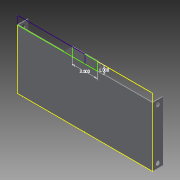
# Autodesk Inventor part: 4barFrontPlate
Saved by Autodesk Inventor 2015 SP1 (Build 190203100, 203)
## iProperties
Created: 2015-02-16
Part Number: 4barFrontPlate
Material: Generic
Document SubType Name: Modeling
Designer: 55221
Density: 1 g/cm^3
Appearance: Default
Author: 55221
Autodesk Inventor part; units mm, degrees
ref_plane "YZ Plane" through (0, 0, 0) normal (1, 0, 0) x (0, 1, 0)
ref_plane "XZ Plane" through (0, 0, 0) normal (0, 1, 0) x (-1, 0, 0)
ref_plane "XY Plane" through (0, 0, 0) normal (0, 0, 1) x (1, 0, 0)
sketch "Sketch1" plane through (0, 0, 0) normal (0, 1, 0) x (-1, 0, 0)
  line L0 (-203.2, 0) -> (203.2, 0)
  line L1 (-200.66, 0) -> (-203.2, 0)
  line L2 (-203.2, 0) -> (-203.2, -22.86)
  line L3 (-200.66, -22.86) -> (-200.66, 0)
  line L4 (203.2, 0) -> (200.66, 0)
  line L5 (203.2, -22.86) -> (203.2, 0)
  arc A0 (-200.66, 2.54) -> (-203.2, 0) centre (-200.66, 0) ccw
  arc A1 (203.2, 0) -> (200.66, 2.54) centre (200.66, 0) ccw
  line L6 (-200.66, 2.54) -> (200.66, 2.54)
  line L7 (200.66, 0) -> (200.66, -29.21)
  line L8 (200.66, -29.21) -> (203.2, -29.21)
  line L9 (203.2, -29.21) -> (203.2, -22.86)
  line L10 (-203.2, 0) -> (-203.2, -29.21)
  line L11 (-203.2, -29.21) -> (-200.66, -29.21)
  line L12 (-200.66, -29.21) -> (-200.66, -22.86)
  line L13 (203.2, 0) -> (200.66, 0)
  point P0 (0, 0)
  dimension "d0" = 406.4
  dimension "d1" = 2.54
  dimension "d5" = 2.54
  dimension "d6" = 2.54
  dimension "d7" = 401.32
  dimension "d8" = 29.21
  dimension "d9" = 29.21
  constraints: 28 end point, 5 perpendicular, 4 point on circle, 3 horizontal, 2 centre point, 2 vertical, 1 collinear, 1 parallel, 1 point on line
  measures "d0" distance of L0.end L0.start
  measures "d1" distance of L3.start L2.end
  measures "d5" radius of A0
  measures "d6" radius of A1
  measures "d7" distance of L6.start L6.end
  measures "d8" distance of L7.start L7.end
  measures "d9" distance of L1.end L10.end
extrude "Extrusion1" add sketch "Sketch1" along normal blind 203.2
sketch "Sketch2" plane through (203.2, 0, 0) normal (1, 0, 0) x (0, 0, -1)
  circle A0 centre (13.97, 12.7) radius 6.35
  circle A1 centre (13.97, 165.1) radius 6.35
  point P0 (0, 0)
  dimension "d12" = 12.7
  dimension "d13" = 12.7
  constraints: 2 centre point
  measures "d12" diameter of A0
  measures "d13" diameter of A1
extrude "Extrusion2" cut sketch "Sketch2" against normal blind 406.4
sketch "Sketch3" plane through (-200.66, 0, 2.54) normal (0, 0, 1) x (1, 0, 0)
  line L0 (-2.54, 0) -> (-2.54, 203.2) projected
  line L1 (0, 203.2) -> (401.32, 203.2) projected
  line L2 (0, 203.2) -> (-2.54, 203.2) projected
  line L3 (403.86, 203.2) -> (401.32, 203.2) projected
  line L4 (403.86, 0) -> (403.86, 203.2) projected
  line L5 (0, 0) -> (401.32, 0) projected
  line L6 (403.86, 0) -> (401.32, 0) projected
  line L7 (0, 0) -> (-2.54, 0) projected
  line L8 (0, 177.8) -> (200.66, 177.8)
  line L9 (200.66, 177.8) -> (200.66, 203.2)
  line L10 (200.66, 203.2) -> (0, 203.2)
  line L11 (0, 177.8) -> (-2.54, 177.8)
  line L12 (-2.54, 177.8) -> (-2.54, 203.2)
  line L13 (-2.54, 203.2) -> (0, 203.2)
  line L14 (162.56, 203.2) -> (238.76, 203.2)
  line L15 (238.76, 203.2) -> (238.76, 177.8)
  line L16 (238.76, 177.8) -> (162.56, 177.8)
  line L17 (162.56, 177.8) -> (162.56, 203.2)
  point P0 (200.66, 0)
  dimension "d16" = 76.2
  dimension "d17" = 25.4
  constraints: 20 end point, 4 parallel, 3 horizontal, 3 perpendicular, 1 midpoint
  measures "d16" distance of L15.end L16.end
  measures "d17" distance of L14.end L15.end
sketch "Sketch4" plane through (-200.66, 0, 2.54) normal (0, 0, 1) x (1, 0, 0)
  line L0 (0, 203.2) -> (401.32, 203.2) projected
  line L1 (162.558, 203.2) -> (198.118, 203.2) construction
  line L2 (264.16, 177.8002) -> (238.76, 177.8002)
  line L3 (238.76, 203.2) -> (264.1598, 177.8002)
  line L4 (264.1598, 177.8002) -> (406.3779, 177.8002)
  line L5 (403.86, 0) -> (403.86, 203.2) projected
  line L6 (403.86, 177.8002) -> (403.86, 203.2)
  line L7 (403.86, 203.2) -> (238.76, 203.2)
  line L8 (162.558, 177.8002) -> (137.158, 177.8002)
  line L9 (137.158, 177.8002) -> (162.558, 203.2)
  line L10 (162.558, 203.2) -> (-2.542, 203.2)
  line L11 (-2.542, 177.8002) -> (-2.542, 203.2)
  line L12 (-2.542, 203.2) -> (162.558, 203.2)
  line L13 (137.158, 177.8002) -> (-2.542, 177.8002)
  line L14 (-2.54, 0) -> (-2.54, 203.2) projected
  point P0 (200.66, 0)
  dimension "d21" = 25.4
  dimension "d22" = 165.1
  constraints: 24 end point, 5 horizontal, 5 point on line, 3 perpendicular, 1 collinear, 1 vertical
  measures "d21" distance of L8.start L8.end
  measures "d22" distance of L1.start L10.end
extrude "Extrusion3" cut sketch "Sketch4" against normal blind 31.75
body "Solid1"
